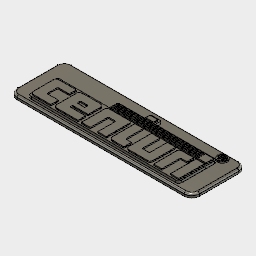
Centuri-WG (Autodesk Fusion 360 design; units mm, degrees)
Autodesk Fusion 360 part; units mm, degrees
sketch "Sketch1" plane through (0, 0, 0) normal (0, 1, 0) x (1, 0, 0)
  arc A0 (143.727, -0.1323) -> (150.0188, -6.4294) centre (143.7217, -6.4294) cw
  line L0 (143.727, -0.1323) -> (6.4294, -0.1323)
  arc A1 (0.1323, -6.4294) -> (6.4294, -0.1323) centre (6.4294, -6.4294) cw
  line L1 (0.1323, -6.4294) -> (0.1323, -38.8064)
  arc A2 (6.4294, -45.1035) -> (0.1323, -38.8064) centre (6.4294, -38.8064) cw
  line L2 (6.4294, -45.1035) -> (143.7217, -45.1035)
  arc A3 (150.0188, -38.8064) -> (143.7217, -45.1035) centre (143.7217, -38.8064) cw
  line L3 (150.0188, -38.8064) -> (150.0188, -6.4267)
  line L4 (150.0188, -6.4267) -> (150.0188, -6.4294)
extrude "Extrude1" add sketch "Sketch1" along normal blind 3.25
fillet "Fillet1" radius 1.5 8 edges at (0.1323, 3.25, 22.6179) (1.9767, 3.25, 43.2591) (75.0755, 3.25, 45.1035) (148.1744, 3.25, 43.2591) (150.0188, 3.25, 22.6166) (148.1753, 3.25, 1.9776) (75.0782, 3.25, 0.1323) (1.9767, 3.25, 1.9767)
sketch "Sketch2" plane through (0, 3.25, 0) normal (0, 1, 0) x (-1, 0, 0)
  line L0 (-1.6323, 6.4294) -> (-1.6323, 38.8064)
  arc A0 (-1.6323, 38.8064) -> (-6.4294, 43.6035) centre (-6.4294, 38.8064) ccw
  line L1 (-6.4294, 43.6035) -> (-143.7217, 43.6035)
  arc A1 (-143.7217, 43.6035) -> (-148.5188, 38.8064) centre (-143.7217, 38.8064) ccw
  line L2 (-148.5188, 38.8064) -> (-148.5188, 6.4267)
  arc A2 (-148.5187, 6.4267) -> (-143.7257, 1.6323) centre (-143.7217, 6.4294) ccw
  line L3 (-143.7257, 1.6323) -> (-6.4294, 1.6323)
  arc A3 (-6.4294, 1.6323) -> (-1.6323, 6.4294) centre (-6.4294, 6.4294) ccw
  spline S0 degree 2 poles (-15.1446, 17.8666) (-22.0892, 17.8666) (-54.3225, 17.8799) knots 0 0 0 1 1 1
  spline S1 degree 2 poles (-54.3225, 17.8799) (-54.671, 17.8975) (-54.951, 17.7762) knots 0 0 0 1 1 1
  spline S2 degree 3 poles (-54.951, 17.7762) (-55.0172, 17.7498) (-55.1672, 17.6263) (-55.2333, 17.4542) knots 0 0 0 0 1 1 1 1
  spline S3 degree 2 poles (-55.2333, 17.4542) (-55.3105, 17.2447) (-55.2973, 16.9801) knots 0 0 0 1 1 1
  line L4 (-55.2973, 16.9801) -> (-55.2973, 12.2496)
  spline S4 degree 3 poles (-55.2973, 12.2496) (-55.2951, 11.7005) (-55.67, 10.8867) (-56.2169, 10.8867) knots 0 0 0 0 1 1 1 1
  spline S5 degree 3 poles (-56.2169, 10.8867) (-59.7212, 10.8823) (-72.3776, 10.8867) (-76.3054, 10.8867) knots 0 0 0 0 1 1 1 1
  spline S6 degree 3 poles (-76.3054, 10.8867) (-76.8567, 10.8867) (-77.1434, 10.9308) (-77.1566, 10.3861) knots 0 0 0 0 1 1 1 1
  spline S7 degree 2 poles (-77.1566, 10.3861) (-77.1853, 9.1754) (-77.1566, 6.8135) knots 0 0 0 1 1 1
  spline S8 degree 3 poles (-77.1566, 6.8135) (-77.1566, 6.4055) (-77.4874, 6.0747) (-77.8954, 6.0747) knots 0 0 0 0 1 1 1 1
  line L5 (-77.8954, 6.0747) -> (-85.1444, 6.0747)
  spline S9 degree 3 poles (-85.1444, 6.0747) (-85.5524, 6.0747) (-85.8832, 6.4055) (-85.8832, 6.8135) knots 0 0 0 0 1 1 1 1
  spline S10 degree 2 poles (-85.8832, 6.8135) (-85.8589, 9.3496) (-85.8743, 10.3707) knots 0 0 0 1 1 1
  spline S11 degree 3 poles (-85.8743, 10.3707) (-85.8832, 10.9441) (-86.2647, 10.8845) (-86.7741, 10.8867) knots 0 0 0 0 1 1 1 1
  spline S12 degree 3 poles (-86.7741, 10.8867) (-94.9339, 10.8978) (-126.5673, 10.8889) (-134.8263, 10.8867) knots 0 0 0 0 1 1 1 1
  spline S13 degree 3 poles (-134.8263, 10.8867) (-135.5695, 10.8867) (-136.251, 11.8571) (-136.251, 12.6025) knots 0 0 0 0 1 1 1 1
  line L6 (-136.251, 12.6025) -> (-136.2576, 20.2837)
  line L7 (-136.2576, 20.2837) -> (-136.2576, 39.6179)
  spline S14 degree 3 poles (-136.2576, 39.6179) (-136.2576, 41.5917) (-135.7945, 42.0328) (-133.8405, 42.0328) knots 0 0 0 0 1 1 1 1
  line L8 (-133.8405, 42.0328) -> (-15.1446, 42.0328)
  spline S15 degree 3 poles (-15.1446, 42.0328) (-13.0584, 42.0328) (-12.4651, 41.6314) (-12.4651, 39.6179) knots 0 0 0 0 1 1 1 1
  line L9 (-12.4651, 39.6179) -> (-12.4651, 20.2837)
  spline S16 degree 3 poles (-12.4651, 20.2837) (-12.4651, 18.2658) (-13.0319, 17.8666) (-15.1446, 17.8666) knots 0 0 0 0 1 1 1 1
extrude "Extrude2" add sketch "Sketch2" along normal blind 2 contours S0 S1 S2 S3 L4 S4 S5 S6 S7 S8 L5 S9 S10 S11 S12 S13 L6 L7 S14 L8 S15 L9 S16
sketch "Sketch4" plane through (0, 5.25, 0) normal (0, 1, 0) x (-1, 0, 0)
  line L0 (-12.4651, 20.2837) -> (-12.4651, 39.6179)
  spline S0 degree 3 poles (-12.4651, 39.6179) (-12.4651, 41.6314) (-13.0584, 42.0328) (-15.1446, 42.0328) knots -1 -1 -1 -1 0 0 0 0
  line L1 (-15.1446, 42.0328) -> (-133.8405, 42.0328)
  spline S1 degree 3 poles (-133.8405, 42.0328) (-135.7945, 42.0328) (-136.2576, 41.5917) (-136.2576, 39.6179) knots -1 -1 -1 -1 0 0 0 0
  line L2 (-136.2576, 39.6179) -> (-136.2576, 20.2837)
  line L3 (-136.2576, 20.2837) -> (-136.251, 12.6025)
  spline S2 degree 3 poles (-136.251, 12.6025) (-136.251, 11.8571) (-135.5695, 10.8867) (-134.8263, 10.8867) knots -1 -1 -1 -1 0 0 0 0
  spline S3 degree 3 poles (-134.8263, 10.8867) (-126.5673, 10.8889) (-94.9339, 10.8978) (-86.7741, 10.8867) knots -1 -1 -1 -1 0 0 0 0
  spline S4 degree 3 poles (-86.7741, 10.8867) (-86.2647, 10.8845) (-85.8832, 10.9441) (-85.8743, 10.3707) knots -1 -1 -1 -1 0 0 0 0
  spline S5 degree 2 poles (-85.8743, 10.3707) (-85.8589, 9.3496) (-85.8832, 6.8135) knots -1 -1 -1 0 0 0
  spline S6 degree 3 poles (-85.8832, 6.8135) (-85.8832, 6.4055) (-85.5524, 6.0747) (-85.1444, 6.0747) knots -1 -1 -1 -1 0 0 0 0
  line L4 (-85.1444, 6.0747) -> (-77.8954, 6.0747)
  spline S7 degree 3 poles (-77.8954, 6.0747) (-77.4874, 6.0747) (-77.1566, 6.4055) (-77.1566, 6.8135) knots -1 -1 -1 -1 0 0 0 0
  spline S8 degree 2 poles (-77.1566, 6.8135) (-77.1853, 9.1754) (-77.1566, 10.3861) knots -1 -1 -1 0 0 0
  spline S9 degree 3 poles (-77.1566, 10.3861) (-77.1434, 10.9308) (-76.8567, 10.8867) (-76.3054, 10.8867) knots -1 -1 -1 -1 0 0 0 0
  spline S10 degree 3 poles (-76.3054, 10.8867) (-72.3776, 10.8867) (-59.7212, 10.8823) (-56.2169, 10.8867) knots -1 -1 -1 -1 0 0 0 0
  spline S11 degree 3 poles (-56.2169, 10.8867) (-55.67, 10.8867) (-55.2951, 11.7005) (-55.2973, 12.2496) knots -1 -1 -1 -1 0 0 0 0
  line L5 (-55.2973, 12.2496) -> (-55.2973, 16.9801)
  spline S12 degree 2 poles (-55.2973, 16.9801) (-55.3105, 17.2447) (-55.2333, 17.4542) knots -1 -1 -1 0 0 0
  spline S13 degree 3 poles (-55.2333, 17.4542) (-55.1672, 17.6263) (-55.0172, 17.7498) (-54.951, 17.7762) knots -1 -1 -1 -1 0 0 0 0
  spline S14 degree 2 poles (-54.951, 17.7762) (-54.671, 17.8975) (-54.3225, 17.8799) knots -1 -1 -1 0 0 0
  spline S15 degree 2 poles (-54.3225, 17.8799) (-22.0892, 17.8666) (-15.1446, 17.8666) knots -1 -1 -1 0 0 0
  spline S16 degree 3 poles (-15.1446, 17.8666) (-13.0319, 17.8666) (-12.4651, 18.2658) (-12.4651, 20.2837) knots -1 -1 -1 -1 0 0 0 0
  spline S17 degree 2 poles (-29.7871, 19.8177) (-18.1613, 19.7975) (-15.4377, 19.8177) knots 0 0 0 1 1 1
  spline S18 degree 3 poles (-15.4377, 19.8177) (-14.4153, 19.8235) (-13.1372, 20.8031) (-13.1314, 21.8116) knots 0 0 0 0 1 1 1 1
  spline S19 degree 3 poles (-13.1314, 21.8116) (-13.1108, 24.9733) (-13.1225, 35.2352) (-13.1314, 38.3911) knots 0 0 0 0 1 1 1 1
  spline S20 degree 3 poles (-13.1314, 38.3911) (-13.1314, 39.5011) (-14.3124, 40.8197) (-15.4377, 40.8226) knots 0 0 0 0 1 1 1 1
  line L6 (-15.4377, 40.8226) -> (-29.7666, 40.8226)
  line L7 (-29.7666, 40.8226) -> (-29.7871, 34.4962)
  spline S21 degree 2 poles (-29.7871, 34.4962) (-22.7329, 34.4904) (-21.1434, 34.4962) knots 0 0 0 1 1 1
  spline S22 degree 3 poles (-21.1434, 34.4962) (-20.6057, 34.4962) (-20.2473, 33.7022) (-20.2532, 33.1689) knots 0 0 0 0 1 1 1 1
  spline S23 degree 3 poles (-20.2532, 33.1689) (-20.2708, 31.9315) (-20.262, 28.2742) (-20.2532, 27.0019) knots 0 0 0 0 1 1 1 1
  spline S24 degree 3 poles (-20.2532, 27.0019) (-20.2532, 26.4948) (-20.6263, 25.7152) (-21.1405, 25.7152) knots 0 0 0 0 1 1 1 1
  line L8 (-21.1405, 25.7152) -> (-29.7871, 25.7152)
  line L9 (-29.7871, 25.7152) -> (-29.7871, 19.8177)
  spline S25 degree 3 poles (-49.6689, 19.8177) (-46.8101, 19.8061) (-37.9167, 19.8033) (-34.9904, 19.8177) knots 0 0 0 0 1 1 1 1
  spline S26 degree 3 poles (-34.9904, 19.8177) (-33.8446, 19.8235) (-32.1846, 20.664) (-32.1904, 21.8) knots 0 0 0 0 1 1 1 1
  spline S27 degree 3 poles (-32.1904, 21.8) (-32.1993, 25.0284) (-32.1904, 35.6148) (-32.1904, 38.7273) knots 0 0 0 0 1 1 1 1
  spline S28 degree 3 poles (-32.1904, 38.7273) (-32.1904, 39.8865) (-33.8211, 40.8197) (-34.9904, 40.8226) knots 0 0 0 0 1 1 1 1
  line L10 (-34.9904, 40.8226) -> (-52.1368, 40.8226)
  line L11 (-52.1368, 40.8226) -> (-52.1368, 34.4962)
  line L12 (-52.1368, 34.4962) -> (-39.6971, 34.4962)
  spline S29 degree 3 poles (-39.6971, 34.4962) (-39.0096, 34.4962) (-39.0096, 32.4589) (-39.6971, 32.4589) knots 0 0 0 0 1 1 1 1
  line L13 (-39.6971, 32.4589) -> (-52.1368, 32.4589)
  line L14 (-52.1368, 32.4589) -> (-52.1368, 21.8)
  spline S30 degree 3 poles (-52.1368, 21.8) (-52.1368, 20.7509) (-50.7266, 19.8207) (-49.6689, 19.8177) knots 0 0 0 0 1 1 1 1
  line L15 (-39.4915, 28.8319) -> (-45.773, 28.8319)
  line L16 (-45.773, 28.8319) -> (-45.773, 26.665)
  spline S31 degree 3 poles (-45.773, 26.665) (-45.773, 26.3973) (-45.4792, 26.1108) (-45.2236, 26.1108) knots 0 0 0 0 1 1 1 1
  line L17 (-45.2236, 26.1108) -> (-40.0673, 26.1108)
  spline S32 degree 3 poles (-40.0673, 26.1108) (-39.8088, 26.1108) (-39.4915, 26.391) (-39.4915, 26.665) knots 0 0 0 0 1 1 1 1
  line L18 (-39.4915, 26.665) -> (-39.4915, 28.8319)
  line L19 (-55.0102, 40.8197) -> (-62.276, 40.8197)
  line L20 (-62.276, 40.8197) -> (-62.276, 27.2077)
  spline S33 degree 3 poles (-62.276, 27.2077) (-62.276, 26.46) (-62.2554, 25.947) (-62.7255, 25.947) knots 0 0 0 0 1 1 1 1
  spline S34 degree 3 poles (-62.7255, 25.947) (-63.651, 25.947) (-66.8887, 25.9413) (-67.8612, 25.947) knots 0 0 0 0 1 1 1 1
  spline S35 degree 3 poles (-67.8612, 25.947) (-68.3989, 25.947) (-68.3989, 26.5035) (-68.3989, 27.2077) knots 0 0 0 0 1 1 1 1
  line L21 (-68.3989, 27.2077) -> (-68.3989, 40.7878)
  line L22 (-68.3989, 40.7878) -> (-75.4002, 40.8226)
  line L23 (-75.4002, 40.8226) -> (-75.4002, 21.8)
  spline S36 degree 3 poles (-75.4002, 21.8) (-75.4002, 20.8987) (-74.4513, 19.8177) (-73.5375, 19.8177) knots 0 0 0 0 1 1 1 1
  spline S37 degree 3 poles (-73.5375, 19.8177) (-70.4203, 19.8177) (-60.2605, 19.812) (-57.1609, 19.8177) knots 0 0 0 0 1 1 1 1
  spline S38 degree 3 poles (-57.1609, 19.8177) (-56.1796, 19.8177) (-55.0102, 20.832) (-55.0102, 21.8) knots 0 0 0 0 1 1 1 1
  line L24 (-55.0102, 21.8) -> (-55.0102, 40.8197)
  line L25 (-77.9828, 19.8177) -> (-84.8872, 19.8177)
  line L26 (-84.8872, 19.8177) -> (-84.8872, 33.7746)
  spline S39 degree 3 poles (-84.8872, 33.7746) (-84.8872, 34.1195) (-85.2868, 34.4962) (-85.6364, 34.4962) knots 0 0 0 0 1 1 1 1
  line L27 (-85.6364, 34.4962) -> (-89.8789, 34.4962)
  line L28 (-89.8789, 34.4962) -> (-89.9259, 40.8255)
  spline S40 degree 2 poles (-89.9259, 40.8255) (-83.2507, 40.8197) (-81.2146, 40.8255) knots 0 0 0 1 1 1
  spline S41 degree 3 poles (-81.2146, 40.8255) (-77.6596, 40.8371) (-77.974, 38.339) (-77.971, 37.0291) knots 0 0 0 0 1 1 1 1
  line L29 (-77.971, 37.0291) -> (-77.9828, 19.8148)
  line L30 (-77.9828, 19.8148) -> (-77.9828, 19.8177)
  line L31 (-91.7034, 19.8177) -> (-98.5696, 19.8177)
  line L32 (-98.5696, 19.8177) -> (-98.5696, 33.7224)
  spline S42 degree 3 poles (-98.5696, 33.7224) (-98.5696, 34.0383) (-98.8047, 34.4933) (-99.1279, 34.4962) knots 0 0 0 0 1 1 1 1
  line L33 (-99.1279, 34.4962) -> (-104.1637, 34.4962)
  spline S43 degree 3 poles (-104.1637, 34.4962) (-104.4634, 34.4962) (-104.6044, 34.018) (-104.6044, 33.7224) knots 0 0 0 0 1 1 1 1
  line L34 (-104.6044, 33.7224) -> (-104.6044, 19.8177)
  line L35 (-104.6044, 19.8177) -> (-111.5617, 19.8177)
  line L36 (-111.5617, 19.8177) -> (-111.5617, 38.4694)
  spline S44 degree 3 poles (-111.5617, 38.4694) (-111.5617, 39.4692) (-110.7537, 40.8226) (-109.649, 40.8226) knots 0 0 0 0 1 1 1 1
  line L37 (-109.649, 40.8226) -> (-93.5779, 40.8226)
  spline S45 degree 3 poles (-93.5779, 40.8226) (-92.5496, 40.8226) (-91.7034, 39.4083) (-91.7034, 38.4694) knots 0 0 0 0 1 1 1 1
  line L38 (-91.7034, 38.4694) -> (-91.7034, 19.8177)
  line L39 (-126.437, 19.8177) -> (-126.437, 25.4834)
  line L40 (-126.437, 25.4834) -> (-122.3237, 25.4834)
  spline S46 degree 3 poles (-122.3237, 25.4834) (-121.7155, 25.4834) (-121.1279, 26.2455) (-121.1279, 26.8483) knots 0 0 0 0 1 1 1 1
  line L41 (-121.1279, 26.8483) -> (-121.1279, 40.8255)
  line L42 (-121.1279, 40.8255) -> (-114.4292, 40.8255)
  line L43 (-114.4292, 40.8255) -> (-114.4292, 21.9797)
  spline S47 degree 3 poles (-114.4292, 21.9797) (-114.4292, 20.7915) (-116.0951, 19.8177) (-117.2997, 19.8177) knots 0 0 0 0 1 1 1 1
  line L44 (-117.2997, 19.8177) -> (-126.437, 19.8177)
  line L45 (-128.2262, 19.8177) -> (-135.1571, 19.8177)
  line L46 (-135.1571, 19.8177) -> (-135.1571, 40.8197)
  line L47 (-135.1571, 40.8197) -> (-128.2233, 40.7501)
  line L48 (-128.2233, 40.7501) -> (-128.2233, 19.8149)
  line L49 (-128.2233, 19.8149) -> (-128.2262, 19.8177)
  arc A0 (-83.9471, 7.4564) -> (-84.4579, 7.965) centre (-83.9493, 7.965) cw
  line L50 (-83.9471, 7.4564) -> (-78.6441, 7.4564)
  arc A1 (-78.1355, 7.965) -> (-78.6441, 7.4564) centre (-78.6441, 7.965) cw
  line L51 (-78.1355, 7.965) -> (-78.1355, 10.5922)
  arc A2 (-78.6441, 11.103) -> (-78.1355, 10.5922) centre (-78.6441, 10.5944) cw
  line L52 (-78.6441, 11.103) -> (-83.9471, 11.103)
  arc A3 (-84.4557, 10.5944) -> (-83.9471, 11.103) centre (-83.9471, 10.5944) cw
  line L53 (-84.4557, 10.5944) -> (-84.4557, 7.965)
  line L54 (-84.4557, 7.965) -> (-84.4579, 7.965)
  line L55 (-56.2604, 12.275) -> (-135.1763, 12.275)
  line L56 (-135.1763, 12.275) -> (-135.1763, 18.6058)
  line L57 (-135.1763, 18.6058) -> (-56.2604, 18.6058)
  spline S48 degree 3 poles (-56.2604, 18.6058) (-55.8491, 18.6058) (-55.8197, 17.6453) (-56.2604, 17.6453) knots 0 0 0 0 1 1 1 1
  line L58 (-56.2604, 17.6453) -> (-128.2131, 17.6453)
  spline S49 degree 3 poles (-128.2131, 17.6453) (-128.8066, 17.6453) (-128.8007, 16.7507) (-128.2131, 16.7536) knots 0 0 0 0 1 1 1 1
  spline S50 degree 3 poles (-128.2131, 16.7536) (-116.22, 16.811) (-68.2212, 16.7622) (-56.2604, 16.7536) knots 0 0 0 0 1 1 1 1
  spline S51 degree 3 poles (-56.2604, 16.7536) (-55.8403, 16.7536) (-55.8491, 15.859) (-56.2604, 15.859) knots 0 0 0 0 1 1 1 1
  line L59 (-56.2604, 15.859) -> (-128.2131, 15.859)
  spline S52 degree 3 poles (-128.2131, 15.859) (-128.833, 15.859) (-128.8007, 14.9673) (-128.2131, 14.9673) knots 0 0 0 0 1 1 1 1
  line L60 (-128.2131, 14.9673) -> (-56.2604, 14.9673)
  spline S53 degree 3 poles (-56.2604, 14.9673) (-55.8374, 14.9673) (-55.8638, 14.0727) (-56.2604, 14.0727) knots 0 0 0 0 1 1 1 1
  spline S54 degree 3 poles (-56.2604, 14.0727) (-68.2594, 14.067) (-116.1818, 14.0727) (-128.2131, 14.0727) knots 0 0 0 0 1 1 1 1
  spline S55 degree 3 poles (-128.2131, 14.0727) (-128.7537, 14.0727) (-128.7566, 13.1782) (-128.2131, 13.1782) knots 0 0 0 0 1 1 1 1
  line L61 (-128.2131, 13.1782) -> (-56.2604, 13.1782)
  spline S56 degree 3 poles (-56.2604, 13.1782) (-55.8403, 13.1782) (-55.8432, 12.275) (-56.2604, 12.275) knots 0 0 0 0 1 1 1 1
extrude "Extrude3" add sketch "Sketch4" along normal blind 1 contours S17 S18 S19 S20 L6 L7 S21 S22 S23 S24 L8 L9 | S25 S26 S27 S28 L10 L11 L12 S29 L13 L14 S30 | L19 L20 S33 S34 S35 L21 L22 L23 S36 S37 S38 L24 | L25 L26 S39 L27 L28 S40 S41 L29 | L31 L32 S42 L33 S43 L34 L35 L36 S44 L37 S45 L38 | L39 L40 S46 L41 L42 L43 S47 L44 | L45 L46 L47 L48 L49 | A0 L50 A1 L51 A2 L52 A3 L53 L54 | L55 L56 L57 S48 L58 S49 S50 S51 L59 S52 L60 S53 S54 S55 L61 S56
sketch "Sketch8" plane through (0, 3.25, 0) normal (0, 1, 0) x (-1, 0, 0)
  spline S0 degree 3 poles (-12.4651, 20.2837) (-12.4651, 18.2658) (-13.0319, 17.8666) (-15.1446, 17.8666) knots 0 0 0 0 1 1 1 1
  spline S1 degree 2 poles (-15.1446, 17.8666) (-22.0892, 17.8666) (-54.3225, 17.8799) knots 0 0 0 1 1 1
  spline S2 degree 2 poles (-54.3225, 17.8799) (-54.671, 17.8975) (-54.951, 17.7762) knots 0 0 0 1 1 1
  spline S3 degree 3 poles (-54.951, 17.7762) (-55.0172, 17.7498) (-55.1672, 17.6263) (-55.2333, 17.4542) knots 0 0 0 0 1 1 1 1
  spline S4 degree 2 poles (-55.2333, 17.4542) (-55.3105, 17.2447) (-55.2973, 16.9801) knots 0 0 0 1 1 1
  line L0 (-55.2973, 16.9801) -> (-55.2973, 12.2496)
  spline S5 degree 3 poles (-55.2973, 12.2496) (-55.2951, 11.7005) (-55.67, 10.8867) (-56.2169, 10.8867) knots 0 0 0 0 1 1 1 1
  spline S6 degree 3 poles (-56.2169, 10.8867) (-59.7212, 10.8823) (-72.3776, 10.8867) (-76.3054, 10.8867) knots 0 0 0 0 1 1 1 1
  spline S7 degree 3 poles (-76.3054, 10.8867) (-76.8567, 10.8867) (-77.1434, 10.9308) (-77.1566, 10.3861) knots 0 0 0 0 1 1 1 1
  spline S8 degree 2 poles (-77.1566, 10.3861) (-77.1853, 9.1754) (-77.1566, 6.8135) knots 0 0 0 1 1 1
  spline S9 degree 3 poles (-77.1566, 6.8135) (-77.1566, 6.4055) (-77.4874, 6.0747) (-77.8954, 6.0747) knots 0 0 0 0 1 1 1 1
  line L1 (-77.8954, 6.0747) -> (-85.1444, 6.0747)
  spline S10 degree 3 poles (-85.1444, 6.0747) (-85.5524, 6.0747) (-85.8832, 6.4055) (-85.8832, 6.8135) knots 0 0 0 0 1 1 1 1
  spline S11 degree 2 poles (-85.8832, 6.8135) (-85.8589, 9.3496) (-85.8743, 10.3707) knots 0 0 0 1 1 1
  spline S12 degree 3 poles (-85.8743, 10.3707) (-85.8832, 10.9441) (-86.2647, 10.8845) (-86.7741, 10.8867) knots 0 0 0 0 1 1 1 1
  spline S13 degree 3 poles (-86.7741, 10.8867) (-94.9339, 10.8978) (-126.5673, 10.8889) (-134.8263, 10.8867) knots 0 0 0 0 1 1 1 1
  spline S14 degree 3 poles (-134.8263, 10.8867) (-135.5695, 10.8867) (-136.251, 11.8571) (-136.251, 12.6025) knots 0 0 0 0 1 1 1 1
  line L2 (-136.251, 12.6025) -> (-136.2576, 20.2837)
  line L3 (-136.2576, 20.2837) -> (-136.2576, 39.6179)
  spline S15 degree 3 poles (-136.2576, 39.6179) (-136.2576, 41.5917) (-135.7945, 42.0328) (-133.8405, 42.0328) knots 0 0 0 0 1 1 1 1
  line L4 (-133.8405, 42.0328) -> (-15.1446, 42.0328)
  spline S16 degree 3 poles (-15.1446, 42.0328) (-13.0584, 42.0328) (-12.4651, 41.6314) (-12.4651, 39.6179) knots 0 0 0 0 1 1 1 1
  line L5 (-12.4651, 39.6179) -> (-12.4651, 20.2837)
  line L6 (-1.6323, 6.4294) -> (-1.6323, 38.8064)
  arc A0 (-1.6323, 38.8064) -> (-6.4294, 43.6035) centre (-6.4294, 38.8064) ccw
  line L7 (-6.4294, 43.6035) -> (-143.7217, 43.6035)
  arc A1 (-143.7217, 43.6035) -> (-148.5188, 38.8064) centre (-143.7217, 38.8064) ccw
  line L8 (-148.5188, 38.8064) -> (-148.5188, 6.4267)
  arc A2 (-148.5187, 6.4267) -> (-143.7257, 1.6323) centre (-143.7217, 6.4294) ccw
  line L9 (-143.7257, 1.6323) -> (-6.4294, 1.6323)
  arc A3 (-6.4294, 1.6323) -> (-1.6323, 6.4294) centre (-6.4294, 6.4294) ccw
  circle A4 centre (-136.3548, 6.1791) radius 4
  circle A5 centre (-136.3548, 6.1791) radius 3.125
  dimension "d11" = 8
  dimension "d12" = 6.25
  measures "d11" diameter of A4
  measures "d12" diameter of A5
extrude "Extrude5" add sketch "Sketch8" along normal blind 1 contours A4
sketch "Sketch9" plane through (0, 3.25, 0) normal (0, 1, 0) x (-1, 0, 0)
  circle A0 centre (-136.3548, 6.1791) radius 3.125
  line L0 (-135.0738, 8.2262) -> (-134.5303, 8.2283)
  line L1 (-134.5303, 8.2283) -> (-134.5368, 4.0057)
  line L2 (-134.5368, 4.0057) -> (-137.5374, 3.9992)
  line L3 (-137.5374, 3.9992) -> (-137.907, 3.9992)
  spline S0 degree 3 poles (-137.907, 3.9992) (-138.1332, 3.9992) (-138.5811, 4.5863) (-138.5941, 5.1777) knots 0 0 0 0 1 1 1 1
  spline S1 degree 3 poles (-138.5941, 5.1777) (-138.6115, 5.9496) (-138.1332, 6.4997) (-137.8962, 6.5041) knots 0 0 0 0 1 1 1 1
  line L4 (-137.8962, 6.5041) -> (-137.5265, 6.4997)
  line L5 (-137.5265, 6.4997) -> (-138.2441, 8.2175)
  line L6 (-138.2441, 8.2175) -> (-137.6961, 8.2175)
  line L7 (-137.6961, 8.2175) -> (-136.9938, 6.4997)
  line L8 (-136.9938, 6.4997) -> (-135.0673, 6.4954)
  line L9 (-135.0673, 6.4954) -> (-135.0738, 8.2262)
  line L10 (-135.076, 4.5102) -> (-137.383, 4.4971)
  line L11 (-137.383, 4.4971) -> (-137.4917, 4.4971)
  spline S2 degree 3 poles (-137.4917, 4.4971) (-137.6179, 4.5015) (-138.0201, 4.6537) (-138.0201, 5.1755) knots 0 0 0 0 1 1 1 1
  spline S3 degree 3 poles (-138.0201, 5.1755) (-138.0201, 5.904) (-137.6287, 5.93) (-137.4917, 5.93) knots 0 0 0 0 1 1 1 1
  line L12 (-137.4917, 5.93) -> (-137.3787, 5.93)
  line L13 (-137.3787, 5.93) -> (-135.0782, 5.9192)
  line L14 (-135.0782, 5.9192) -> (-135.0782, 4.5102)
  line L15 (-135.0782, 4.5102) -> (-135.076, 4.5102)
extrude "Extrude6" add sketch "Sketch9" along normal blind 1 contours L0 L1 L2 L3 S0 S1 L4 L5 L6 L7 L8 L9
